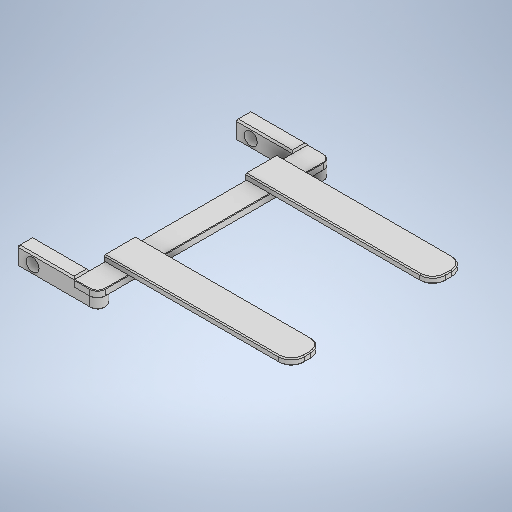
# Autodesk Inventor part: Fork
Saved by Autodesk Inventor 2025.2 (Build 292293000, 293)
## iProperties
Created: 2025-02-20
Part Number: Fork
Material: Generic
Document SubType Name: Modeling
Designer: Sergio Quintero
Density: 1 g/cm^3
Appearance: Default
Author: Sergio Quintero
Autodesk Inventor part; units mm, degrees
ref_plane "YZ Plane" through (0, 0, 0) normal (1, 0, 0) x (0, 1, 0)
ref_plane "XZ Plane" through (0, 0, 0) normal (0, 1, 0) x (-1, 0, 0)
ref_plane "XY Plane" through (0, 0, 0) normal (0, 0, 1) x (1, 0, 0)
sketch "Sketch1" plane through (0, 0, 0) normal (0, 1, 0) x (-1, 0, 0)
  line L0 (-55, -15) -> (55, -15)
  line L1 (55, -15) -> (55, 15)
  line L2 (55, 15) -> (-55, 15)
  line L3 (-55, 15) -> (-55, -15)
  line L4 (-55, -15) -> (55, 15) construction
  line L5 (55, -15) -> (-55, 15) construction
  point P0 (0, 0)
  dimension "d0" = 110
  dimension "d1" = 30
  constraints: 12 end point, 2 midpoint, 2 parallel, 1 horizontal, 1 perpendicular
  measures "d0" distance of L2.end L1.end
  measures "d1" distance of L1.end L0.end
extrude "Extrusion1" add sketch "Sketch1" along normal blind 36
sketch "Sketch2" plane through (55, 0, 15) normal (1, 0, 0) x (0, 0, -1)
  line L0 (30, 0) -> (0, 0) projected
  line L1 (30, 0) -> (30, 36) projected
  line L2 (0, 0) -> (30, 0)
  line L3 (30, 0) -> (30, 21)
  line L4 (30, 21) -> (0, 21)
  line L5 (0, 21) -> (0, 0)
  point P0 (15, 0)
  dimension "d4" = 21
  constraints: 8 end point, 2 parallel, 1 horizontal, 1 perpendicular, 1 point on line
  measures "d4" distance between parallel lines of L0 L4
extrude "Extrusion2" add sketch "Sketch2" along normal blind 45
fillet "Fillet1" radius 15 1 edges at (100, 10.5, 15)
fillet "Fillet2" radius 15 1 edges at (100, 10.5, -15)
chamfer "Chamfer1" distance 3 angle 45 12 edges at (0, 36, 15) (-55, 36, 0) (0, 36, -15) (55, 36, 0) (15, 0, 15) (100, 0, -0.0001) (95.6066, 0, -10.6066) (95.6066, 0, 10.6066) (15.0001, 0, -15) (-55, 0, 0) (-55, 18, -15) (-55, 18, 15)
sketch "Sketch3" plane through (55, 21, 15) normal (0, 1, 0) x (1, 0, 0)
  line L0 (0, 0) -> (30, 0) projected
  line L1 (0, 0) -> (45, 0)
  line L2 (45, 0) -> (45, 450)
  line L3 (45, 450) -> (0, 450)
  line L4 (0, 450) -> (0, 0)
  point P0 (-55, 15)
  dimension "d12" = 45
  dimension "d13" = 450
  constraints: 8 end point, 2 parallel, 1 horizontal, 1 perpendicular
  measures "d12" distance of L3.end L2.end
  measures "d13" distance of L2.end L1.end
extrude "Extrusion3" add sketch "Sketch3" along normal blind 12 separate body
fillet "Fillet3" radius 15 1 edges at (100, 27, 15)
fillet "Fillet4" radius 15 1 edges at (100, 27, -435)
sketch "Sketch4" plane through (55, 33, 15) normal (0, 1, 0) x (1, 0, 0)
  line L0 (0, 0) -> (0, 450)
  line L1 (0, 58) -> (360, 58)
  line L2 (360, 58) -> (360, 120)
  line L3 (360, 120) -> (0, 120)
  line L4 (0, 120) -> (0, 58)
  line L5 (30, 0) -> (0, 0)
  point P0 (-55, 15)
  point P1 (360, 89)
  point P2 (0, 120)
  dimension "d18" = 360
  dimension "d19" = 62
  dimension "d20" = 58
  constraints: 12 end point, 2 parallel, 1 horizontal, 1 midpoint, 1 perpendicular, 1 point on line
  measures "d18" distance from line of point (360, 89) L0
  measures "d19" distance between parallel lines of L3 L1
  measures "d20" distance between parallel lines of L5 L1
extrude "Extrusion4" add sketch "Sketch4" along normal blind 12 separate body
fillet "Fillet5" radius 25 1 edges at (415, 39, -43)
fillet "Fillet6" radius 25 1 edges at (415, 39, -105)
chamfer "Chamfer2" distance 2 angle 45 5 edges at (222.5, 45, -43) (407.6777, 45, -50.3223) (415, 45, -74) (407.6777, 45, -97.6777) (222.5, 45, -105)
chamfer "Chamfer3" distance 2 angle 45 5 edges at (222.5, 33, -43) (407.6777, 33, -50.3223) (415, 33, -74) (407.6777, 33, -97.6777) (222.5, 33, -105)
chamfer "Chamfer4" distance 1 angle 45 6 edges at (95.6066, 33, 10.6066) (85, 33, 15) (70, 33, 15) (100, 33, -209.9999) (95.6066, 33, -430.6066) (70, 33, -435)
ref_plane "Work Plane1" through (55, 21, -210) normal (0, 0, 1) x (1, 0, 0)
mirror "Mirror1" about plane through (55, 21, -210) normal (0, 0, 1) of "Extrusion1", "Extrusion2", "Fillet1", "Fillet2", "Chamfer1", "Extrusion4", "Fillet5", "Fillet6", "Chamfer2", "Chamfer3" bodies 1
sketch "Sketch5" plane through (55, 21, 15) normal (0, 0, 1) x (1, 0, 0)
  circle A0 centre (-80, -3) radius 12.5
  line L0 (-110, 12) -> (-110, -18) projected
  line L1 (-3, 15) -> (-107, 15) projected
  point P0 (-55, -21)
  dimension "d34" = 25
  dimension "d35" = 30
  dimension "d36" = 18
  constraints: 1 centre point
  measures "d34" diameter of A0
  measures "d35" distance from line of L0 A0.centre
  measures "d36" distance from line of L1 A0.centre
extrude "Extrusion5" cut sketch "Sketch5" against normal up to surface (450 mm away) bodies 1
body "Solid1"
body "Solid2"
body "Solid3"
